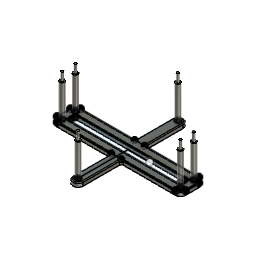
stand_veh v3 (Autodesk Fusion 360 design; units mm, degrees)
Autodesk Fusion 360 part; units mm, degrees
sketch "Sketch1" plane through (0, 0, 0) normal (0, 0, 1) x (1, 0, 0)
  line L0 (-3, 0) -> (-6, 0)
  line L1 (-77, 52) -> (-77, 68)
  line L2 (77, 52) -> (77, 68)
  line L3 (44.954, 74) -> (71, 74)
  line L4 (44.954, 74) -> (6, 74)
  line L5 (44.954, 46) -> (6, 46)
  line L6 (44.954, 46) -> (71, 46)
  line L7 (-44.954, 74) -> (-6, 74)
  line L8 (-44.954, 46) -> (-6, 46)
  line L9 (-44.954, 74) -> (-71, 74)
  line L10 (-44.954, 46) -> (-71, 46)
  line L11 (6, 0) -> (6, 46)
  line L12 (-6, 0) -> (-6, 46)
  line L13 (-6, 120) -> (-6, 74)
  line L14 (6, 120) -> (6, 74)
  arc A0 (-71, 74) -> (-77, 68) centre (-71, 68) ccw
  arc A1 (-77, 52) -> (-71, 46) centre (-71, 52) ccw
  arc A2 (6, 120) -> (-6, 120) centre (0, 120) ccw
  arc A3 (77, 68) -> (71, 74) centre (71, 68) ccw
  arc A4 (71, 46) -> (77, 52) centre (71, 52) ccw
  arc A5 (-6, 0) -> (6, 0) centre (0, 0) ccw
  dimension "d7" = 12
  dimension "d8" = 12
  dimension "d12" = 46
  constraint perpendicular L0 L1
  constraint tangent L11 A5
  constraint perpendicular L5 L11
  measures "d7" diameter of A2
  measures "d8" diameter of A3
  measures "d12" distance of L11.start L5.end
extrude "Extrude1" add sketch "Sketch1" along normal blind 5
sketch "Sketch2" plane through (0, 0, 5) normal (0, 0, 1) x (-1, 0, 0)
  line L0 (71, -46) -> (6, -46)
  line L1 (6, -46) -> (6, 0)
  arc A0 (6, 0) -> (-6, 0) centre (0, 0) ccw
  line L2 (-6, 0) -> (-6, -46)
  line L3 (-6, -46) -> (-71, -46)
  arc A1 (-71, -46) -> (-77, -52) centre (-71, -52) ccw
  line L4 (-77, -52) -> (-77, -68)
  arc A2 (-77, -68) -> (-71, -74) centre (-71, -68) ccw
  line L5 (-71, -74) -> (-6, -74)
  line L6 (-6, -74) -> (-6, -120)
  arc A3 (-6, -120) -> (6, -120) centre (0, -120) ccw
  line L7 (6, -120) -> (6, -74)
  line L8 (6, -74) -> (71, -74)
  arc A4 (71, -74) -> (77, -68) centre (71, -68) ccw
  line L9 (77, -68) -> (77, -52)
  arc A5 (77, -52) -> (71, -46) centre (71, -52) ccw
  circle A6 centre (0, -120) radius 3
  circle A7 centre (0, -120) radius 1.5
  line L10 (0, 0) -> (0, -60)
  line L11 (0, -60) -> (-26, -60)
  circle A8 centre (0, 0) radius 1.5
  circle A9 centre (0, 0) radius 3
  circle A10 centre (-71, -68) radius 3
  circle A11 centre (-71, -68) radius 1.5
  circle A12 centre (-71, -52) radius 3
  circle A13 centre (-71, -52) radius 1.5
  circle A14 centre (71, -68) radius 3
  circle A15 centre (71, -68) radius 1.5
  circle A16 centre (71, -52) radius 3
  circle A17 centre (71, -52) radius 1.5
  line L12 (-6, -46) -> (6, -46)
  line L13 (-6, -74) -> (6, -74)
  line L14 (-6, -46) -> (-71, -46)
  line L15 (-77, -52) -> (-77, -68)
  line L16 (-71, -74) -> (-6, -74)
  line L17 (6, -46) -> (71, -46)
  line L18 (77, -52) -> (77, -68)
  line L19 (71, -74) -> (6, -74)
  arc A18 (77, -52) -> (71, -46) centre (71, -52) ccw
  arc A19 (71, -74) -> (77, -68) centre (71, -68) ccw
  arc A20 (-71, -46) -> (-77, -52) centre (-71, -52) ccw
  arc A21 (-77, -68) -> (-71, -74) centre (-71, -68) ccw
  arc A22 (-71, -46) -> (-77, -52) centre (-71, -52) ccw
  arc A23 (-77, -68) -> (-71, -74) centre (-71, -68) ccw
  line L20 (68, -57.5) -> (68, -62.5)
  line L21 (65.5, -65) -> (6, -65)
  line L22 (-6, -65) -> (6, -65)
  line L23 (-65.5, -65) -> (-6, -65)
  line L24 (-68, -57.5) -> (-68, -62.5)
  line L25 (-6, -55) -> (-65.5, -55)
  line L26 (-6, -55) -> (6, -55)
  line L27 (6, -55) -> (65.5, -55)
  arc A24 (-65.5, -55) -> (-68, -57.5) centre (-65.5, -57.5) ccw
  arc A25 (-68, -62.5) -> (-65.5, -65) centre (-65.5, -62.5) ccw
  arc A26 (68, -57.5) -> (65.5, -55) centre (65.5, -57.5) ccw
  arc A27 (65.5, -65) -> (68, -62.5) centre (65.5, -62.5) ccw
  dimension "d15" = 6
  dimension "d16" = 3
  dimension "d17" = 60
  dimension "d18" = 6
  dimension "d19" = 3
  dimension "d28" = 12
  dimension "d30" = 2.5
  dimension "d31" = 2.5
  constraint concentric A3 A6
  constraint concentric A6 A7
  constraint coincident A0.centre L10.start
  constraint parallel L2 L10
  constraint perpendicular L2 L11
  constraint symmetric A6 L11 A9
  constraint symmetric A7 L11 A8
  constraint concentric A2 A10
  constraint concentric A10 A11
  constraint symmetric L11 A10 A12
  constraint symmetric L11 A11 A13
  constraint symmetric L10 A10 A14
  constraint symmetric L10 A11 A15
  constraint symmetric L10 A12 A16
  constraint symmetric L10 A13 A17
  constraint concentric A12 A22
  constraint symmetric L11 A21 A22
  constraint symmetric L11 A22 A23
  constraint symmetric L11 A20 A21
  constraint coincident L2.end L3.start
  constraint coincident L0.end L1.start
  constraint coincident L5.end L6.start
  constraint coincident L7.end L8.start
  constraint coincident L3.end A1.start
  constraint coincident A1.end L4.start
  constraint coincident L4.end A2.start
  constraint coincident A2.end L5.start
  constraint coincident L0.start A5.end
  constraint symmetric L10 A18 A22
  constraint symmetric L10 A19 A21
  constraint coincident L9.end A5.start
  constraint coincident A4.end L9.start
  constraint coincident L8.end A4.start
  constraint tangent L24 A24
  constraint tangent L25 A24
  constraint tangent L23 A25
  constraint tangent L24 A25
  constraint equal A24 A25
  constraint tangent L20 A26
  constraint tangent L27 A26
  constraint equal A24 A26
  constraint tangent L20 A27
  constraint tangent L21 A27
  measures "d15" diameter of A6
  measures "d16" diameter of A7
  measures "d17" distance of A0.centre L10.end
  measures "d18" diameter of A10
  measures "d19" diameter of A11
  measures "d28" diameter of A22
  measures "d30" radius of A24
  measures "d31" radius of A27
extrude "Extrude2" add sketch "Sketch2" along normal blind 50 contours A7 | A8 | A11 | A13 | A15 | A17
extrude "Extrude3" add sketch "Sketch2" along normal blind 40 contours A6 | A9 | A10 | A12 | A14 | A16
fillet "Fillet1" radius 2.5 4 edges at (6, 46, 2.5) (-6, 46, 2.5) (-6, 74, 2.5) (6, 74, 2.5)
fillet "Fillet2" radius 1 20 edges at (6.7322, 74.7322, 5) (6, 98.25, 5) (0, 126, 5) (-6, 98.25, 5) (-6.7322, 74.7322, 5) (-39.75, 74, 5) (-75.2426, 72.2426, 5) (-77, 60, 5) (-75.2426, 47.7574, 5) (-39.75, 46, 5) (-6.7322, 45.2678, 5) (-6, 21.75, 5) (0, -6, 5) (6, 21.75, 5) (6.7322, 45.2678, 5) (39.75, 46, 5) (75.2426, 47.7574, 5) (77, 60, 5) (75.2426, 72.2426, 5) (39.75, 74, 5)
extrude "Extrude4" cut sketch "Sketch2" against normal blind 14 contours L20 L21 L22 L23 L24 L25 L26 L27 A24 A25 A26 A27
fillet "Fillet3" radius 1 8 edges at (-68, 60, 5) (-67.2678, 64.2678, 5) (0, 65, 5) (67.2678, 64.2678, 5) (68, 60, 5) (67.2678, 55.7322, 5) (0, 55, 5) (-67.2678, 55.7322, 5)
